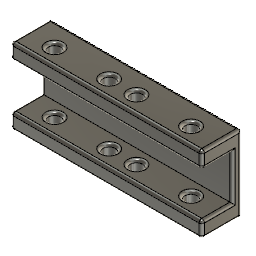
railConnector (Autodesk Fusion 360 design; units mm, degrees)
Autodesk Fusion 360 part; units mm, degrees
sketch "Sketch1" plane through (0, 0, 0) normal (0, 1, 0) x (1, 0, 0)
  line L0 (-35, -14) -> (35, -14)
  line L1 (35, -14) -> (35, 14)
  line L2 (35, 14) -> (-35, 14)
  line L3 (-35, 14) -> (-35, -14)
  line L4 (-35, -14) -> (35, 14) construction
  line L5 (35, -14) -> (-35, 14) construction
  dimension "d1" = 70
  dimension "d2" = 28
  constraint horizontal L0
  constraint perpendicular L0 L1
  constraint parallel L0 L2
  constraint parallel L1 L3
  constraint coincident L4 origin
  constraint coincident L5 origin
  measures "d1" distance of L1.end L2.end
  measures "d2" distance of L0.end L1.end
extrude "Extrude1" add sketch "Sketch1" along normal blind 16
sketch "Sketch2" plane through (0, 0, 0) normal (0, -1, 0) x (1, 0, 0)
  line L0 (-35, 14) -> (-35, -14)
  line L1 (-35, -14) -> (35, -14)
  line L2 (35, -14) -> (35, 14)
  line L3 (35, 14) -> (-35, 14)
  line L4 (-35, 8.15) -> (35, 8.15)
  line L5 (35, 8.15) -> (35, -8.15)
  line L6 (35, -8.15) -> (-35, -8.15)
  line L7 (-35, -8.15) -> (-35, 8.15)
  line L8 (-35, 8.15) -> (35, -8.15) construction
  line L9 (35, 8.15) -> (-35, -8.15) construction
  dimension "d5" = 70
  dimension "d6" = 16.3
  constraint horizontal L4
  constraint perpendicular L4 L5
  constraint parallel L4 L6
  constraint parallel L5 L7
  constraint coincident L8 origin
  constraint coincident L9 origin
  measures "d5" distance of L5.end L6.end
  measures "d6" distance of L4.end L5.end
extrude "Extrude2" cut sketch "Sketch2" against normal blind 11.3 contours L0 L2 L4 L5 L6 L7
sketch "Sketch3" plane through (0, 0, 14) normal (0, 0, 1) x (-1, 0, 0)
  line L0 (35, 0) -> (-35, 0)
  line L1 (-35, 0) -> (-35, -16)
  line L2 (-35, -16) -> (35, -16)
  line L3 (35, -16) -> (35, 0)
  circle A0 centre (-5, -6.1) radius 2.25
  line L4 (35, -11.3) -> (-35, -11.3)
  circle A1 centre (-25, -6.1) radius 2.25
  line L5 (0, -1.75) -> (0, -22.5)
  circle A2 centre (25, -6.1) radius 2.25
  circle A3 centre (5, -6.1) radius 2.25
  dimension "d9" = 4.5
  dimension "d10" = 5.2
  dimension "d11" = 5
  dimension "d12" = 4.5
  dimension "d13" = 20
  dimension "d14" = 5.2
  constraint symmetric A0 L5 A3
  constraint symmetric A1 L5 A2
  measures "d9" diameter of A0
  measures "d10" distance of A0.centre L4
  measures "d11" horizontal distance of origin A0.centre
  measures "d12" diameter of A1
  measures "d13" horizontal distance of A0.centre A1.centre
  measures "d14" distance of L4 A1.centre
extrude "Extrude3" cut sketch "Sketch3" against normal blind 40 contours A0 | A1 | A2 | A3
chamfer "Chamfer1" distance 2 angle 45 1 faces at (-11.6667, 16, -4.6667)
fillet "Fillet1" radius 1 10 edges at (0, 0, -8.15) (0, 0, 8.15) (-22.9023, 5.2864, -8.15) (-2.9023, 5.2864, -8.15) (7.0977, 5.2864, -8.15) (27.0977, 5.2864, -8.15) (27.0977, 6.9136, 8.15) (7.0977, 6.9136, 8.15) (-2.9023, 6.9136, 8.15) (-22.9023, 6.9136, 8.15) 4 faces at (-32.4083, 6.8118, 14) (-32.4083, 6.8118, -14) (35, 8.4333, -12.05) (-35, 8.4333, -12.05)
